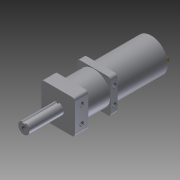
# Autodesk Inventor part: Banebot P60 20to1 with RS-550 Motor
Saved by Autodesk Inventor 2013 (Build 170138000, 138)
## iProperties
Created: 2012-01-28
Part Number: Banebot P60 20to1 with RS-550 Motor
Document SubType Name: Modeling
Designer: niemitalo_dan
Density: 3.64745 g/cm^3
Mass: 453.592 g
Surface Area: 211.827 cm^2
Volume: 124.359 cm^3
Material: Generic
Author: niemitalo_dan
Autodesk Inventor part; units mm, degrees
ref_plane "YZ Plane" through (0, 0, 0) normal (1, 0, 0) x (0, 1, 0)
ref_plane "XZ Plane" through (0, 0, 0) normal (0, 1, 0) x (-1, 0, 0)
sketch "Sketch3" plane through (0, 0, 0) normal (0, 0, 1) x (1, 0, 0)
  line L0 (-19.05, 19.05) -> (19.05, 19.05)
  line L1 (19.05, 19.05) -> (19.05, -19.05)
  line L2 (19.05, -19.05) -> (-19.05, -19.05)
  line L3 (-19.05, -19.05) -> (-19.05, 19.05)
  point P0 (0, 0)
  point P1 (-19.05, 0)
  point P2 (0, 19.05)
  dimension "d4" = 38.1
  dimension "d5" = 38.1
  constraints: 8 end point, 2 midpoint, 2 parallel, 1 horizontal, 1 horizontal alignment, 1 perpendicular, 1 vertical alignment
  measures "d4" distance of L1.end L2.end
  measures "d5" distance of L0.end L1.end
extrude "Extrusion2" add sketch "Sketch3" along normal blind 7.62
sketch "Sketch4" plane through (0, 0, 7.62) normal (0, 0, 1) x (1, 0, 0)
  circle A0 centre (0, 0) radius 18.415
  dimension "d8" = 36.83
  constraints: 1 centre point, 1 coincident
  measures "d8" diameter of A0
extrude "Extrusion3" add sketch "Sketch4" along normal blind 25.4
sketch "Sketch5" plane through (0, 0, 33.02) normal (0, 0, 1) x (1, 0, 0)
  circle A0 centre (0, 0) radius 18.415 projected
  line L0 (19.05, 19.05) -> (19.05, -19.05) projected
  line L1 (-19.05, 19.05) -> (19.05, 19.05) projected
  line L2 (-19.05, -19.05) -> (-19.05, 19.05) projected
  line L3 (19.05, -19.05) -> (-19.05, -19.05) projected
extrude "Extrusion4" add sketch "Sketch5" along normal blind 15.24 contours A0 | L0 L3 L2 L1
sketch "Sketch6" plane through (0, 0, 48.26) normal (0, 0, 1) x (1, 0, 0)
  circle A0 centre (0, 0) radius 6.35
  line L0 (-1.5875, 7.7359) -> (1.5875, 7.7359)
  line L1 (1.5875, 7.7359) -> (1.5875, 4.5609)
  line L2 (1.5875, 4.5609) -> (-1.5875, 4.5609)
  line L3 (-1.5875, 4.5609) -> (-1.5875, 7.7359)
  line L4 (-1.5875, 6.1484) -> (1.5875, 6.1484) construction
  point P0 (0, 0)
  point P1 (0, 4.5609)
  dimension "d13" = 12.7
  dimension "d14" = 3.175
  dimension "d16" = 1.5875
  constraints: 10 end point, 3 midpoint, 2 parallel, 2 point on circle, 1 centre point, 1 coincident, 1 horizontal, 1 perpendicular, 1 vertical alignment
  measures "d13" diameter of A0
  measures "d14" distance of L0.start L0.end
  measures "d16" distance between parallel lines of L2 L4
extrude "Extrusion5" add sketch "Sketch6" along normal blind 38.608 contours A0 L3 L2 L1 picked at (0.1781, 0.9314)
sketch "Sketch7" plane through (19.05, -19.05, 33.02) normal (1, 0, 0) x (0, 0, -1)
  line L0 (0, 0) -> (-15.24, 0) projected
  line L1 (0, 38.1) -> (-15.24, 38.1) projected
  line L2 (25.4, 38.1) -> (25.4, 0) projected
  line L3 (33.02, 0) -> (25.4, 0) projected
  line L4 (33.02, 38.1) -> (33.02, 0) projected
  line L5 (33.02, 38.1) -> (25.4, 38.1) projected
  point P0 (33.02, 19.05)
  point P1 (-7.62, 28.575)
  point P2 (-7.62, 9.525)
  point P3 (-7.62, 38.1)
  point P4 (-7.62, 0)
  point P5 (29.21, 28.575)
  point P6 (29.21, 9.525)
  point P7 (29.21, 38.1)
  point P8 (29.21, 0)
  dimension "d19" = 9.525
  dimension "d20" = 9.525
  constraints: 4 midpoint, 4 vertical alignment, 2 horizontal alignment
  measures "d19" distance from line of L1 point (-7.62, 28.575)
  measures "d20" distance from line of L0 point (-7.62, 9.525)
hole "Hole1" at (19.05, 9.525, 40.64) at (19.05, -9.525, 40.64) at (19.05, 9.525, 3.81) at (19.05, -9.525, 3.81) direction (-1, 0, 0) diameter 4.9784 depth 25.4 tip angle 118 thread size "1/4-20 UNC" class "2B" standard "ANSI Unified Screw Threads"
ref_plane "Work Plane1" through (0, -19.05, 33.02) normal (1, 0, 0) x (0, 0, -1)
mirror "Mirror1" about plane through (0, -19.05, 33.02) normal (1, 0, 0) of "Hole1"
sketch "Sketch8" plane through (0, 0, 86.868) normal (0, 0, 1) x (1, 0, 0)
  arc A0 (-1.5875, 6.1484) -> (1.5875, 6.1484) centre (0, 0) ccw projected
  constraints: 1 coincident
hole "Hole2" at (0, 0, 86.868) direction (0, 0, -1) diameter 4.9784 depth 25.4 tip angle 118 thread size "1/4-20 UNC" class "2B" standard "ANSI Unified Screw Threads"
sketch "Sketch9" plane through (0, 0, 0) normal (0, 0, -1) x (-1, 0, 0)
  circle A0 centre (0, 0) radius 18.669
  dimension "d35" = 37.338
  constraints: 1 centre point, 1 coincident
  measures "d35" diameter of A0
extrude "Extrusion6" add sketch "Sketch9" along normal blind 57.15
sketch "Sketch10" plane through (0, 0, -57.15) normal (0, 0, -1) x (-1, 0, 0)
  circle A0 centre (0, 0) radius 18.669 projected
  line L0 (-14.605, 1.905) -> (-13.97, 1.905)
  line L1 (-13.97, 1.905) -> (-13.97, -1.905)
  line L2 (-13.97, -1.905) -> (-14.605, -1.905)
  line L3 (-14.605, -1.905) -> (-14.605, 1.905)
  line L4 (13.97, 1.905) -> (14.605, 1.905)
  line L5 (14.605, 1.905) -> (14.605, -1.905)
  line L6 (14.605, -1.905) -> (13.97, -1.905)
  line L7 (13.97, -1.905) -> (13.97, 1.905)
  point P0 (-13.97, 0)
  point P1 (13.97, 0)
  dimension "d38" = 3.81
  dimension "d39" = 0.635
  dimension "d40" = 13.97
  dimension "d41" = 13.97
  constraints: 16 end point, 4 parallel, 2 equal length, 2 horizontal, 2 horizontal alignment, 2 midpoint, 2 perpendicular
  measures "d38" distance of L2.end L0.start
  measures "d39" distance of L0.start L0.end
  measures "d40" distance from line of A0.centre L1
  measures "d41" distance from line of L7 A0.centre
extrude "Extrusion7" add sketch "Sketch10" along normal blind 5.461 separate body contours L0 L1 L2 L3 | L4 L5 L6 L7
sketch "Sketch11" plane through (0, 0, -57.15) normal (0, 0, -1) x (-1, 0, 0)
  circle A0 centre (0, 0) radius 18.669 projected
  circle A1 centre (0, 0) radius 6.35
  dimension "d44" = 12.7
  constraints: 1 centre point, 1 coincident
  measures "d44" diameter of A1
extrude "Extrusion8" add sketch "Sketch11" along normal blind 4.064 contours A1 bodies 1
sketch "Sketch12" plane through (0, 0, -61.214) normal (0, 0, -1) x (-1, 0, 0)
  circle A0 centre (0, 0) radius 6.35 projected
  circle A1 centre (0, 0) radius 1.6
  dimension "d47" = 3.2
  constraints: 1 centre point, 1 coincident
  measures "d47" diameter of A1
extrude "Extrusion9" add sketch "Sketch12" along normal blind 1.27 contours A1 bodies 1
fillet "Fillet1" radius 1.5875 1 edges at (6.35, 0, -61.214)
fillet "Fillet2" radius 0.7937 1 edges at (1.6, 0, -62.484)
fillet "Fillet3" radius 3.175 8 edges at (-19.05, 19.05, 3.81) (-19.05, 19.05, 40.64) (-19.05, -19.05, 40.64) (-19.05, -19.05, 3.81) (19.05, 19.05, 3.81) (19.05, 19.05, 40.64) (19.05, -19.05, 3.81) (19.05, -19.05, 40.64)
body "Solid2"
body "Solid3"
